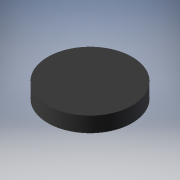
# Autodesk Inventor part: CF Insert Flange Support 01
Saved by Autodesk Inventor 2019 (Build 230136000, 136)
## iProperties
Created: 2019-04-12
Part Number: CF Insert Flange Support 01
Material: Generic
Document SubType Name: Modeling
Designer: isadmin
Density: 1 g/cm^3
Appearance: Default
Author: isadmin
Autodesk Inventor part; units mm, degrees
ref_plane "YZ Plane" through (0, 0, 0) normal (1, 0, 0) x (0, 1, 0)
ref_plane "XZ Plane" through (0, 0, 0) normal (0, 1, 0) x (-1, 0, 0)
ref_plane "XY Plane" through (0, 0, 0) normal (0, 0, 1) x (1, 0, 0)
sketch "Sketch1" plane through (0, 0, 0) normal (0, 0, 1) x (1, 0, 0)
  line L0 (-34.925, -12.7) -> (0, -12.7)
  line L1 (0, -12.7) -> (0, 0)
  line L2 (0, 0) -> (-34.925, 0)
  line L3 (-34.925, 0) -> (-34.925, -12.7)
  line L4 (-34.925, 0) -> (0, 0)
  line L5 (0, 0) -> (0, -12.7)
  dimension "d0" = 34.925
  dimension "d1" = 12.7
  constraints: 12 end point, 4 perpendicular, 1 collinear, 1 horizontal
  measures "d0" distance of L0.end L0.start
  measures "d1" distance of L2.end L0.start
revolve "Revolution1" add sketch "Sketch1" angle 360 about axis through (0, 0, 0) along (0, -1, 0)
body "Solid1"
